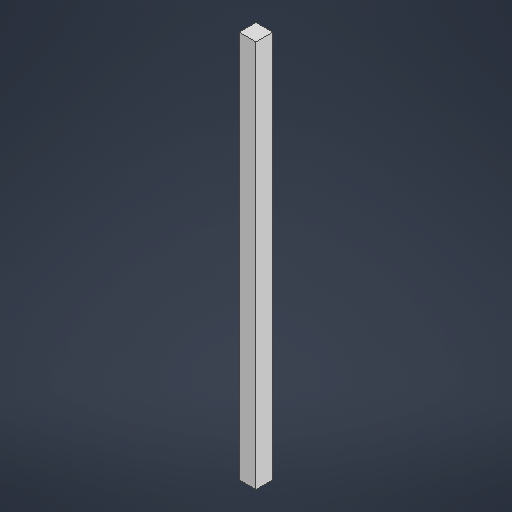
# Autodesk Inventor part: led-wire-long
Saved by Autodesk Inventor 2025.2 (Build 292293000, 293)
## iProperties
Created: 2025-12-13
Part Number: led-wire-long
Material: Generic
Document SubType Name: Modeling
Designer: sam
Density: 1 g/cm^3
Appearance: Default
Author: sam
Autodesk Inventor part; units mm, degrees
ref_plane "YZ Plane" through (0, 0, 0) normal (1, 0, 0) x (0, 1, 0)
ref_plane "XZ Plane" through (0, 0, 0) normal (0, 1, 0) x (-1, 0, 0)
ref_plane "XY Plane" through (0, 0, 0) normal (0, 0, 1) x (1, 0, 0)
sketch "Sketch1" plane through (0, 0, 0) normal (0, 1, 0) x (-1, 0, 0)
  line L0 (0.25, 0.25) -> (-0.25, 0.25)
  line L1 (-0.25, 0.25) -> (-0.25, -0.25)
  line L2 (-0.25, -0.25) -> (0.25, -0.25)
  line L3 (0.25, -0.25) -> (0.25, 0.25)
  line L4 (0.25, 0.25) -> (-0.25, -0.25) construction
  line L5 (-0.25, 0.25) -> (0.25, -0.25) construction
  point P0 (0, 0)
  dimension "d0" = 0.5
  dimension "d1" = 0.5
  constraints: 12 end point, 2 midpoint, 2 parallel, 1 horizontal, 1 perpendicular
  measures "d0" distance of L2.end L1.end
  measures "d1" distance of L1.end L0.end
extrude "Extrusion1" add sketch "Sketch1" along normal blind 11.5
body "Solid1"
